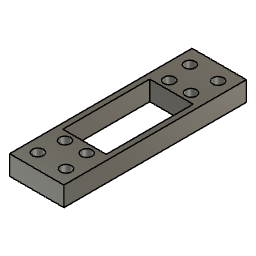
Pos33 (Autodesk Fusion 360 design; units mm, degrees)
Autodesk Fusion 360 part; units mm, degrees
sketch "Sketch1" plane through (0, 0, 0) normal (0, 0, 1) x (1, 0, 0)
  line L0 (12.5, -42) -> (-12.5, -42)
  line L1 (-12.5, -42) -> (-12.5, 42)
  line L2 (-12.5, 42) -> (12.5, 42)
  line L3 (12.5, 42) -> (12.5, -42)
  line L4 (12.5, -42) -> (-12.5, 42) construction
  line L5 (-12.5, -42) -> (12.5, 42) construction
  line L6 (10, -20) -> (-10, -20)
  line L7 (-10, -20) -> (-10, 20)
  line L8 (-10, 20) -> (10, 20)
  line L9 (10, 20) -> (10, -20)
  line L10 (10, -20) -> (-10, 20) construction
  line L11 (-10, -20) -> (10, 20) construction
  circle A0 centre (5, -24) radius 2.5
  circle A1 centre (-5, -24) radius 2.5
  line L12 (0, 0) -> (5, 0) construction
  circle A2 centre (5, 24) radius 2.5
  circle A3 centre (-5, 24) radius 2.5
  circle A4 centre (6.5, 35) radius 2.5
  circle A5 centre (-6.5, 35) radius 2.5
  circle A6 centre (6.5, -35) radius 2.5
  circle A7 centre (-6.5, -35) radius 2.5
  dimension "d1" = 84
  dimension "d2" = 25
  dimension "d3" = 40
  dimension "d4" = 20
  dimension "d5" = 5
  dimension "d6" = 5
  dimension "d7" = 18
  dimension "d8" = 18
  dimension "d9" = 5
  dimension "d10" = 10
  dimension "d11" = 5
  dimension "d12" = 5
  dimension "d13" = 6
  dimension "d14" = 7
  dimension "d15" = 13
  dimension "d16" = 7
  constraint horizontal L0
  constraint perpendicular L0 L1
  constraint parallel L0 L2
  constraint parallel L1 L3
  constraint coincident L4 L12.start
  constraint coincident L5 L12.start
  constraint coincident L12.start origin
  constraint horizontal L6
  constraint perpendicular L6 L7
  constraint parallel L6 L8
  constraint parallel L7 L9
  constraint coincident L10 L12.start
  constraint coincident L11 L12.start
  constraint horizontal L12
  constraint symmetric A0 L12 A2
  constraint symmetric A1 L12 A3
  constraint symmetric L12 A4 A6
  constraint symmetric L12 A5 A7
  measures "d1" distance of L0.start L2.end
  measures "d2" distance of L1.end L2.end
  measures "d3" distance of L6.start L8.end
  measures "d4" distance of L7.end L8.end
  measures "d5" diameter of A0
  measures "d6" diameter of A1
  measures "d7" distance of L0 A0.centre
  measures "d8" distance of L0 A1.centre
  measures "d9" horizontal distance of L12.start A1.centre
  measures "d10" distance of A0.centre A1.centre
  measures "d11" diameter of A4
  measures "d12" diameter of A5
  measures "d13" distance of L3 A4.centre
  measures "d14" distance of L2 A4.centre
  measures "d15" horizontal distance of A4.centre A5.centre
  measures "d16" distance of L2 A5.centre
extrude "Extrude1" add sketch "Sketch1" along normal blind 9
